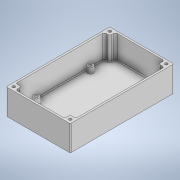
# Autodesk Inventor part: Enclosure Box
Saved by Autodesk Inventor 2021 (Build 250183000, 183)
## iProperties
Created: 2021-06-04
Part Number: Enclosure Box
Material: Generic
Document SubType Name: Modeling
Designer: Anton
Density: 1 g/cm^3
Appearance: Default
Author: Anton
Autodesk Inventor part; units mm, degrees
ref_plane "YZ Plane" through (0, 0, 0) normal (1, 0, 0) x (0, 1, 0)
ref_plane "XZ Plane" through (0, 0, 0) normal (0, 1, 0) x (-1, 0, 0)
ref_plane "XY Plane" through (0, 0, 0) normal (0, 0, 1) x (1, 0, 0)
sketch "Sketch2" plane through (0, 0, 0) normal (0, 1, 0) x (-1, 0, 0)
  line L0 (0, 0) -> (62, 0)
  line L1 (62, 0) -> (62, -66)
  line L2 (62, -66) -> (0, -66)
  line L3 (0, -66) -> (0, 0)
  circle A0 centre (58.15, -9.3) radius 1.5
  circle A1 centre (57.35, -60.86) radius 1.5
  circle A2 centre (3, -4.5) radius 1.5
  circle A3 centre (3, -61.9) radius 1.5
  circle A4 centre (3, -4.5) radius 3
  circle A5 centre (58.15, -9.3) radius 3
  circle A6 centre (57.35, -60.86) radius 3
  circle A7 centre (3, -61.9) radius 3
  line L4 (63, 20) -> (-1, 20)
  line L5 (-1, 20) -> (-1, -86)
  line L6 (-1, -86) -> (63, -86)
  line L7 (63, -86) -> (63, 20)
  dimension "d14" = 66
  dimension "d15" = 62
  dimension "d16" = 3
  dimension "d17" = 3
  dimension "d18" = 3
  dimension "d19" = 3
  dimension "d20" = 3
  dimension "d21" = 4.5
  dimension "d22" = 6
  dimension "d23" = 3
  dimension "d24" = 57.4
  dimension "d25" = 54.35
  dimension "d26" = 0.8
  dimension "d27" = 51.56
  dimension "d28" = 4.8
  dimension "d29" = 6
  dimension "d30" = 6
  dimension "d31" = 6
  dimension "d32" = 20
  dimension "d33" = 20
  dimension "d34" = 1
  dimension "d35" = 1
  constraints: 16 end point, 8 centre point, 4 coincident, 4 parallel, 2 horizontal, 2 perpendicular
  measures "d14" distance between parallel lines of L2 L0
  measures "d15" distance between parallel lines of L3 L1
  measures "d16" diameter of A0
  measures "d17" diameter of A1
  measures "d18" diameter of A3
  measures "d19" diameter of A2
  measures "d20" distance from line of L3 A2.centre
  measures "d21" distance from line of A2.centre L0
  measures "d22" diameter of A4
  measures "d23" distance from line of L3 A3.centre
  measures "d24" distance of A2.centre A3.centre
  measures "d25" horizontal distance of A1.centre A3.centre
  measures "d26" horizontal distance of A1.centre A0.centre
  measures "d27" vertical distance of A1.centre A0.centre
  measures "d28" vertical distance of A2.centre A0.centre
  measures "d29" diameter of A5
  measures "d30" diameter of A6
  measures "d31" diameter of A7
  measures "d32" distance between parallel lines of L4 L0
  measures "d33" distance between parallel lines of L2 L6
  measures "d34" distance between parallel lines of L7 L1
  measures "d35" distance between parallel lines of L3 L5
extrude "Extrusion1" add sketch "Sketch2" along normal blind 2 contours A4 | A7 | L0 L1 L2 L3 | A0 | A1 | A2 | A3 | A5 | A6 | L7 L6 L5 L4
sketch "Sketch4" plane through (0, 2, 0) normal (0, 1, 0) x (1, 0, 0)
  line L0 (-62, 66) -> (0, 66)
  line L1 (0, 66) -> (0, 0)
  line L2 (0, 0) -> (-62, 0)
  line L3 (-62, 0) -> (-62, 66)
  circle A0 centre (-3.85, 56.7) radius 1.5
  circle A1 centre (-4.65, 5.14) radius 1.5
  circle A2 centre (-59, 61.5) radius 1.5
  circle A3 centre (-59, 4.1) radius 1.5
  circle A4 centre (-59, 61.5) radius 3
  circle A5 centre (-3.85, 56.7) radius 3
  circle A6 centre (-4.65, 5.14) radius 3
  circle A7 centre (-59, 4.1) radius 3
  line L4 (1, 86) -> (-63, 86)
  line L5 (-63, 86) -> (-63, -20)
  line L6 (-63, -20) -> (1, -20)
  line L7 (1, -20) -> (1, 86)
  line L8 (1, 86) -> (-63, 86) projected
  line L9 (-63, 86) -> (-63, -20) projected
  point P0 (0, 0)
  dimension "d38" = 66
  dimension "d39" = 62
  dimension "d40" = 3
  dimension "d41" = 3
  dimension "d42" = 3
  dimension "d43" = 3
  dimension "d44" = 3
  dimension "d45" = 4.5
  dimension "d46" = 6
  dimension "d47" = 3
  dimension "d48" = 57.4
  dimension "d49" = 54.35
  dimension "d50" = 0.8
  dimension "d51" = 51.56
  dimension "d52" = 4.8
  dimension "d53" = 6
  dimension "d54" = 6
  dimension "d55" = 6
  dimension "d56" = 20
  dimension "d57" = 20
  dimension "d58" = 1
  dimension "d59" = 1
  dimension "d60" = 0
  dimension "d61" = 0
  constraints: 16 end point, 8 centre point, 4 coincident, 4 parallel, 2 horizontal, 2 perpendicular
  measures "d38" distance between parallel lines of L2 L0
  measures "d39" distance between parallel lines of L3 L1
  measures "d40" diameter of A0
  measures "d41" diameter of A1
  measures "d42" diameter of A3
  measures "d43" diameter of A2
  measures "d44" distance from line of L3 A2.centre
  measures "d45" distance from line of A2.centre L0
  measures "d46" diameter of A4
  measures "d47" distance from line of L3 A3.centre
  measures "d48" distance of A2.centre A3.centre
  measures "d49" horizontal distance of A1.centre A3.centre
  measures "d50" horizontal distance of A1.centre A0.centre
  measures "d51" vertical distance of A1.centre A0.centre
  measures "d52" vertical distance of A2.centre A0.centre
  measures "d53" diameter of A5
  measures "d54" diameter of A6
  measures "d55" diameter of A7
  measures "d56" distance between parallel lines of L4 L0
  measures "d57" distance between parallel lines of L2 L6
  measures "d58" distance between parallel lines of L7 L1
  measures "d59" distance between parallel lines of L3 L5
  measures "d60" distance between parallel lines of L8 L4
  measures "d61" distance between parallel lines of L9 L5
extrude "Extrusion2" add sketch "Sketch4" along normal blind 6 contours A4 | A7 | A5 | A6
sketch "Sketch5" plane through (1, 0, 20) normal (1, 0, 0) x (0, 0, -1)
  line L0 (106, 2) -> (0, 2) projected
  line L1 (36, 2) -> (36, 4)
  line L2 (36, 4) -> (32, 4)
  line L3 (32, 4) -> (32, 2)
  line L4 (69, 2) -> (69, 4)
  line L5 (69, 4) -> (65, 4)
  line L6 (65, 4) -> (65, 2)
  line L7 (71, 2) -> (71, 6)
  line L8 (71, 6) -> (63, 6)
  line L9 (63, 6) -> (63, 2)
  line L10 (38, 2) -> (38, 6)
  line L11 (38, 6) -> (30, 6)
  line L12 (30, 6) -> (30, 2)
  line L13 (30, 2) -> (32, 2)
  line L14 (36, 2) -> (38, 2)
  line L15 (63, 2) -> (65, 2)
  line L16 (69, 2) -> (71, 2)
  line L17 (0, 0) -> (0, 2) projected
  line L18 (106, 0) -> (106, 2) projected
  point P0 (20, 0)
  point P1 (69, 2)
  dimension "d64" = 2
  dimension "d65" = 0
  dimension "d66" = 2
  dimension "d67" = 2
  dimension "d68" = 30
  dimension "d69" = 4
  dimension "d70" = 4
  dimension "d71" = 4
  dimension "d72" = 2
  dimension "d73" = 2
  dimension "d74" = 2
  dimension "d75" = 2
  dimension "d76" = 35
  constraints: 32 end point, 8 parallel, 4 horizontal, 4 perpendicular, 4 point on line
  measures "d64" distance between parallel lines of L11 L2
  measures "d65" distance between parallel lines of L0 L14
  measures "d66" distance between parallel lines of L10 L1
  measures "d67" distance between parallel lines of L12 L3
  measures "d68" distance between parallel lines of L17 L12
  measures "d69" distance between parallel lines of L1 L3
  measures "d70" distance between parallel lines of L0 L11
  measures "d71" distance between parallel lines of L4 L6
  measures "d72" distance between parallel lines of L4 L7
  measures "d73" distance between parallel lines of L9 L6
  measures "d74" distance between parallel lines of L8 L5
  measures "d75" distance between parallel lines of L0 L5
  measures "d76" distance between parallel lines of L18 L7
extrude "Extrusion3" add sketch "Sketch5" against normal blind 8 contours L0 L4 L5 L6 L9 L8 L7 | L0 L1 L2 L3 L12 L11 L10
sketch "Sketch6" plane through (1, 0, 20) normal (1, 0, 0) x (0, 0, -1)
  line L0 (106, 2) -> (0, 2) projected
  line L1 (29.1739, 2) -> (71.7255, 2)
  line L2 (71.7255, 2) -> (71.7255, 7.2821)
  line L3 (71.7255, 7.2821) -> (29.1739, 7.2821)
  line L4 (29.1739, 7.2821) -> (29.1739, 2)
  point P0 (20, 0)
  constraints: 8 end point, 2 parallel, 1 horizontal, 1 perpendicular, 1 point on line
extrude "Extrusion4" cut sketch "Sketch6" against normal blind 4
fillet "Fillet1" radius 1 2 edges at (-5, 4, -45) (-5, 4, -49)
fillet "Fillet2" radius 1 2 edges at (-5, 4, -12) (-5, 4, -16)
fillet "Fillet3" radius 1 8 edges at (-7, 6, -14) (-5, 6, -10) (-3, 6, -14) (-5, 6, -18) (-5, 6, -43) (-3, 6, -47) (-5, 6, -51) (-7, 6, -47)
sketch "Sketch8" plane through (0, 2, 0) normal (0, 1, 0) x (1, 0, 0)
  line L0 (-65, -22) -> (3, -22)
  line L1 (3, -22) -> (3, 88)
  line L2 (3, 88) -> (-65, 88)
  line L3 (-65, 88) -> (-65, -22)
  line L4 (-63, 86) -> (-63, -20) projected
  line L5 (-63, -20) -> (1, -20) projected
  line L6 (1, 86) -> (-63, 86) projected
  line L7 (1, -20) -> (1, 86) projected
  line L8 (-63, -20) -> (1, -20)
  line L9 (1, -20) -> (1, 86)
  line L10 (1, 86) -> (-63, 86)
  line L11 (-63, 86) -> (-63, -20)
  point P0 (0, 0)
  dimension "d86" = 2
  dimension "d87" = 2
  dimension "d88" = 2
  dimension "d89" = 2
  constraints: 16 end point, 4 parallel, 2 horizontal, 2 perpendicular
  measures "d86" distance between parallel lines of L4 L3
  measures "d87" distance between parallel lines of L5 L0
  measures "d88" distance between parallel lines of L6 L2
  measures "d89" distance between parallel lines of L7 L1
extrude "Extrusion5" add sketch "Sketch8" along normal blind 25 and the other way blind 2
fillet "Fillet4" radius 1 4 edges at (3, 13.5, -88) (-65, 13.5, -88) (-65, 13.5, 22) (3, 13.5, 22)
sketch "Sketch9" plane through (0, 2, 0) normal (0, 1, 0) x (1, 0, 0)
  circle A0 centre (-1, 84) radius 1.5
  circle A1 centre (-1, -18) radius 1.5
  circle A2 centre (-61, -18) radius 1.5
  circle A3 centre (-61, 84) radius 1.5
  arc A4 (-58.1277, 86) -> (-63, 81.1277) centre (-61, 84) ccw
  arc A5 (1, 81.1277) -> (-3.8723, 86) centre (-1, 84) ccw
  arc A6 (-3.8723, -20) -> (1, -15.1277) centre (-1, -18) ccw
  arc A7 (-63, -15.1277) -> (-58.1277, -20) centre (-61, -18) ccw
  line L0 (-65, 87) -> (-65, -21) projected
  line L1 (2, 88) -> (-64, 88) projected
  line L2 (3, -21) -> (3, 87) projected
  line L3 (-64, -22) -> (2, -22) projected
  line L4 (1, 86) -> (1, -20) projected
  line L5 (-63, 86) -> (1, 86) projected
  line L6 (1, 86) -> (-5, 86)
  line L7 (-5, 86) -> (-5, 80)
  line L8 (-5, 80) -> (1, 80)
  line L9 (1, 80) -> (1, 86)
  line L10 (1, -20) -> (-63, -20) projected
  line L11 (1, -20) -> (-5, -20)
  line L12 (-5, -20) -> (-5, -14)
  line L13 (-5, -14) -> (1, -14)
  line L14 (1, -14) -> (1, -20)
  line L15 (-63, -20) -> (-63, 86) projected
  line L16 (-63, -20) -> (-57, -20)
  line L17 (-57, -20) -> (-57, -14)
  line L18 (-57, -14) -> (-63, -14)
  line L19 (-63, -14) -> (-63, -20)
  line L20 (-63, 86) -> (-57, 86)
  line L21 (-57, 86) -> (-57, 80)
  line L22 (-57, 80) -> (-63, 80)
  line L23 (-63, 80) -> (-63, 86)
  point P0 (0, 0)
  point P1 (1, -14)
  point P2 (1, 80)
  dimension "d95" = 3
  dimension "d96" = 3
  dimension "d97" = 3
  dimension "d98" = 3
  dimension "d99" = 7
  dimension "d100" = 7
  dimension "d101" = 7
  dimension "d102" = 7
  dimension "d103" = 4
  dimension "d104" = 4
  dimension "d105" = 4
  dimension "d106" = 4
  dimension "d107" = 4
  dimension "d108" = 4
  dimension "d109" = 4
  dimension "d110" = 4
  dimension "d111" = 6
  dimension "d112" = 6
  dimension "d113" = 6
  dimension "d114" = 6
  dimension "d115" = 6
  dimension "d116" = 6
  constraints: 32 end point, 11 point on line, 8 centre point, 8 parallel, 8 point on circle, 4 coincident, 4 horizontal, 4 perpendicular
  measures "d95" diameter of A1
  measures "d96" diameter of A0
  measures "d97" diameter of A3
  measures "d98" diameter of A2
  measures "d99" diameter of A5
  measures "d100" diameter of A6
  measures "d101" diameter of A7
  measures "d102" diameter of A4
  measures "d103" distance from line of L0 A3.centre
  measures "d104" distance from line of L1 A3.centre
  measures "d105" distance from line of L1 A0.centre
  measures "d106" distance from line of L2 A0.centre
  measures "d107" distance from line of L3 A6.centre
  measures "d108" distance from line of L2 A1.centre
  measures "d109" distance from line of L3 A2.centre
  measures "d110" distance from line of L0 A2.centre
  measures "d111" distance of L6.end L7.end
  measures "d112" distance of L7.end L8.end
  measures "d113" distance of L20.end L21.end
  measures "d114" distance of L21.end L22.end
  measures "d115" distance of L16.end L17.end
  measures "d116" distance of L17.end L18.end
extrude "Extrusion6" add sketch "Sketch9" along normal blind 25 contours L5 L21 L22 L15 | L5 L4 L8 L7 | L18 L17 L10 L15 | L4 L10 L12 L13
fillet "Fillet5" radius 2 8 edges at (1, 14.5, 14) (-5, 14.5, 20) (-63, 14.5, 14) (-57, 14.5, 20) (-63, 14.5, -80) (-57, 14.5, -86) (-5, 14.5, -86) (1, 14.5, -80)
fillet "Fillet6" radius 2 4 edges at (-57, 14.5, -80) (-5, 14.5, -80) (-5, 14.5, 14) (-57, 14.5, 14)
fillet "Fillet7" radius 1 24 edges at (-56.4142, 2, -85.4142) (-57, 2, -83) (-57.5858, 2, -80.5858) (-60, 2, -80) (-62.4142, 2, -79.4142) (-63, 2, -33) (-62.4142, 2, 13.4142) (-60, 2, 14) (-57.5858, 2, 14.5858) (-57, 2, 17) (-56.4142, 2, 19.4142) (-31, 2, 20) (-5.5858, 2, 19.4142) (-5, 2, 17) (-4.4142, 2, 14.5858) (-2, 2, 14) (0.4142, 2, 13.4142) (1, 2, -33) (0.4142, 2, -79.4142) (-2, 2, -80) (-4.4142, 2, -80.5858) (-5, 2, -83) (-5.5858, 2, -85.4142) (-31, 2, -86)
body "Solid1"
